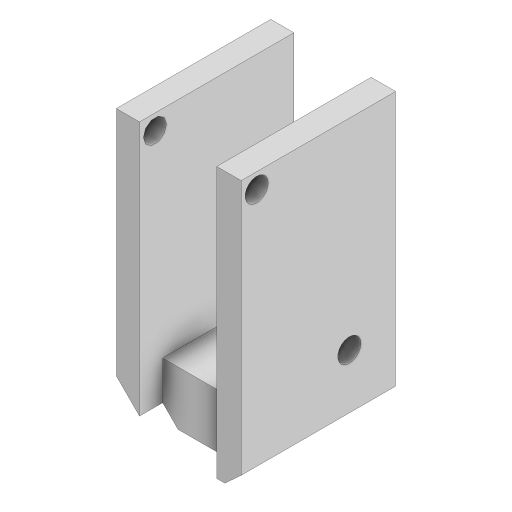
# Autodesk Inventor part: IMPRIMIR SOPORTE
Saved by Autodesk Inventor 2024 (Build 280153000, 153)
## iProperties
Created: 2024-07-19
Part Number: IMPRIMIR SOPORTE
Material: Generic
Document SubType Name: Modeling
Designer: Jhuliams
Density: 1 g/cm^3
Appearance: Default
Author: Jhuliams
Autodesk Inventor part; units mm, degrees
ref_plane "YZ Plane" through (0, 0, 0) normal (1, 0, 0) x (0, 1, 0)
ref_plane "XZ Plane" through (0, 0, 0) normal (0, 1, 0) x (-1, 0, 0)
ref_plane "XY Plane" through (0, 0, 0) normal (0, 0, 1) x (1, 0, 0)
sketch "Sketch1" plane through (0, 0, 0) normal (0, 0, 1) x (1, 0, 0)
  circle A0 centre (0, 0) radius 57.5
  line L0 (0, 0) -> (0, 22.225)
  circle A1 centre (0, 0) radius 60.5
  line L1 (60.5, 0) -> (60.5, 20)
  line L2 (60.5, 0) -> (80.5, 0) construction
  line L3 (-60.5, 0) -> (-60.5, 20)
  line L4 (-60.5, 0) -> (-40.5, 0) construction
  line L5 (-76.5, 37.5) -> (-44.5, 37.5)
  line L6 (-44.5, 37.5) -> (-44.5, 2.5)
  line L7 (-44.5, 2.5) -> (-76.5, 2.5)
  line L8 (-76.5, 2.5) -> (-76.5, 37.5)
  line L9 (-76.5, 37.5) -> (-44.5, 2.5) construction
  line L10 (-44.5, 37.5) -> (-76.5, 2.5) construction
  line L11 (44.5, 37.5) -> (76.5, 37.5)
  line L12 (76.5, 37.5) -> (76.5, 2.5)
  line L13 (76.5, 2.5) -> (44.5, 2.5)
  line L14 (44.5, 2.5) -> (44.5, 37.5)
  line L15 (44.5, 37.5) -> (76.5, 2.5) construction
  line L16 (76.5, 37.5) -> (44.5, 2.5) construction
  point P0 (-57.4456, 2.5)
  point P1 (57.4456, 2.5)
  point P2 (47.4763, 37.5)
  point P3 (-47.4763, 37.5)
  dimension "d0" = 115
  dimension "d27" = 121
  dimension "d28" = 20
  dimension "d29" = 90
  dimension "d30" = 20
  dimension "d31" = 90
  dimension "d32" = 32
  dimension "d33" = 35
  dimension "d34" = 32
  dimension "d35" = 35
  constraints: 34 end point, 4 horizontal, 4 midpoint, 4 parallel, 4 perpendicular, 3 coincident, 3 vertical, 2 centre point, 2 point on circle, 1 tangent
  measures "d0" diameter of A0
  measures "d27" diameter of A1
  measures "d28" distance of L1.start L1.end
  measures "d29" angle of L2 L1
  measures "d30" distance of L3.start L3.end
  measures "d31" angle of L4 L3
  measures "d32" distance of L6.end L7.end
  measures "d33" distance of L5.end L6.end
  measures "d34" distance of L12.end L13.end
  measures "d35" distance of L11.end L12.end
extrude "Extrusion1" add sketch "Sketch1" along normal mid plane 20 contours A0 L14 L11 A1 L13 | L7 A1 L5 L6 A0 | A0 L6 L5 A1 L11 L14 | A1 L11 L12 L13 | L7 L8 L5 A1
sketch "Sketch5" plane through (-76.5, 37.5, 10) normal (0, 1, 0) x (1, 0, 0)
  line L0 (0, 0) -> (0, 20) projected
  line L1 (0, 10) -> (3, 10)
  line L2 (3, 10) -> (8, 10)
  line L3 (13, -5) -> (3, -5)
  line L4 (3, -5) -> (3, 25)
  line L5 (3, 25) -> (13, 25)
  line L6 (13, 25) -> (13, -5)
  line L7 (13, -5) -> (3, 25) construction
  line L8 (3, -5) -> (13, 25) construction
  point P0 (76.5, 10)
  dimension "d36" = 3
  dimension "d37" = 5
  dimension "d38" = 10
  dimension "d39" = 30
  constraints: 16 end point, 3 midpoint, 2 horizontal, 2 parallel, 1 perpendicular, 1 point on line
  measures "d36" distance of L1.start L1.end
  measures "d37" distance of L1.end L2.end
  measures "d38" distance of L4.end L5.end
  measures "d39" distance of L3.end L4.end
extrude "Extrusion5" cut sketch "Sketch5" against normal blind 13
sketch "Sketch6" plane through (-76.5, 24.5, 10) normal (0, 1, 0) x (1, 0, 0)
  line L0 (13, 0) -> (3, 0) projected
  line L1 (13, 20) -> (13, 0) projected
  line L2 (3, 20) -> (13, 20) projected
  line L3 (3, 0) -> (3, 20) projected
  line L4 (8, 0) -> (8, 8)
  line L5 (13, 0) -> (3, 0)
  line L6 (3, 0) -> (3, 16)
  line L7 (3, 16) -> (13, 16)
  line L8 (13, 16) -> (13, 0)
  line L9 (13, 0) -> (3, 16) construction
  line L10 (3, 0) -> (13, 16) construction
  point P0 (76.5, 10)
  dimension "d42" = 8
  dimension "d43" = 10
  dimension "d44" = 16
  constraints: 14 end point, 3 midpoint, 2 parallel, 1 horizontal, 1 perpendicular, 1 vertical
  measures "d42" distance of L4.start L4.end
  measures "d43" distance of L6.end L7.end
  measures "d44" distance of L5.end L6.end
extrude "Extrusion6" cut sketch "Sketch6" against normal blind 15 contours L0 L3 L7 L1
sketch "Sketch7" plane through (-76.5, 2.5, 10) normal (-1, 0, 0) x (0, 0, 1)
  line L0 (0, 35) -> (0, 0) projected
  line L1 (-16, 7) -> (0, 7) projected
  line L2 (0, 35) -> (-16, 35)
  line L3 (-16, 35) -> (-16, 7)
  line L4 (-16, 7) -> (0, 7)
  line L5 (0, 7) -> (0, 35)
  line L6 (-16, 7) -> (-14, 7)
  line L7 (-14, 7) -> (-14, 9)
  line L8 (0, 35) -> (-2, 35)
  line L9 (0, 35) -> (-20, 35) projected
  line L10 (0, 35) -> (2, 35) construction
  line L11 (-2, 35) -> (-2, 33)
  circle A0 centre (-2, 33) radius 1.5
  circle A1 centre (-14, 9) radius 1.5
  point P0 (-10, -2.5)
  dimension "d47" = 16
  dimension "d48" = 28
  dimension "d49" = 2
  dimension "d50" = 2
  dimension "d51" = 90
  dimension "d52" = 2
  dimension "d53" = 180
  dimension "d54" = 2
  dimension "d55" = 3
  dimension "d56" = 3
  constraints: 18 end point, 3 parallel, 2 centre point, 2 coincident, 2 collinear, 2 horizontal, 2 perpendicular, 1 point on line
  measures "d47" distance of L4.end L1.start
  measures "d48" distance of L1.start L2.end
  measures "d49" distance of L1.start L6.end
  measures "d50" distance of L6.end L7.end
  measures "d51" angle of L7 L6
  measures "d52" distance of L0.start L8.end
  measures "d53" angle of L8 L10
  measures "d54" distance of L8.end L11.end
  measures "d55" diameter of A0
  measures "d56" diameter of A1
extrude "Extrusion7" cut sketch "Sketch7" against normal blind 20 contours A0 | A1
mirror "Mirror2" about plane through (0, 0, 0) normal (1, 0, 0) of "Extrusion5", "Extrusion6", "Extrusion7"
chamfer "Chamfer1" distance 5 angle 45 2 edges at (-76.5, 2.5, 0) (76.5, 2.5, 0)
fillet "Fillet1" radius 7 2 edges at (-47.4763, 37.5, 0) (47.4763, 37.5, 0)
chamfer "Chamfer2" distance 5 angle 45 2 edges at (-57.4456, 2.5, 0) (57.4456, 2.5, 0)
sketch "Sketch8" plane through (-76.5, 9.5, 10) normal (0, 1, 0) x (1, 0, 0)
  line L0 (13, 0) -> (3, 0) projected
  line L1 (8, 0) -> (8, 3)
  line L2 (13, 6) -> (3, 6)
  line L3 (3, 6) -> (3, 0)
  line L4 (3, 0) -> (13, 0)
  line L5 (13, 0) -> (13, 6)
  line L6 (13, 6) -> (3, 0) construction
  line L7 (3, 6) -> (13, 0) construction
  line L8 (13, 3) -> (3, 3)
  point P0 (76.5, 10)
  dimension "d66" = 3
  dimension "d67" = 10
  dimension "d68" = 6
  constraints: 16 end point, 5 midpoint, 2 parallel, 1 horizontal, 1 perpendicular, 1 vertical
  measures "d66" distance of L1.start L1.end
  measures "d67" distance of L4.end L0.end
  measures "d68" distance of L0.end L2.end
extrude "Extrusion8" cut sketch "Sketch8" against normal blind 20 contours L0 L1 L8 L5 | L0 L3 L8 L1
mirror "Mirror3" about plane through (0, 0, 0) normal (1, 0, 0) of "Extrusion8"
sketch "Sketch9" plane through (0, 0, 10) normal (0, 0, 1) x (1, 0, 0)
  line L0 (-60.325, 74.6125) -> (82.55, 74.6125)
  line L1 (82.55, 74.6125) -> (82.55, -23.8125)
  line L2 (82.55, -23.8125) -> (-60.325, -23.8125)
  line L3 (-60.325, -23.8125) -> (-60.325, 74.6125)
  point P0 (0, 0)
  constraints: 8 end point, 2 parallel, 1 horizontal, 1 perpendicular
extrude "Extrusion9" cut sketch "Sketch9" against normal blind 30
body "Solid1"
